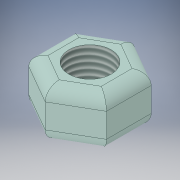
# Autodesk Inventor part: BASE_TUERCA
Saved by Autodesk Inventor 2019 (Build 230136000, 136)
## iProperties
Created: 2020-02-12
Part Number: BASE_TUERCA
Material: Genérico
Document SubType Name: Modeling
Designer: omar-
Density: 1 g/cm^3
Appearance: Valor por defecto
Author: omar-
Autodesk Inventor part; units mm, degrees
ref_plane "YZ Plane" through (0, 0, 0) normal (1, 0, 0) x (0, 1, 0)
ref_plane "XZ Plane" through (0, 0, 0) normal (0, 1, 0) x (-1, 0, 0)
ref_plane "XY Plane" through (0, 0, 0) normal (0, 0, 1) x (1, 0, 0)
sketch "Boceto1" plane through (0, 0, 0) normal (0, 1, 0) x (-1, 0, 0)
  line L0 (0, -7.3901) -> (-6.4, -3.695)
  line L1 (-6.4, -3.695) -> (-6.4, 3.695)
  line L2 (-6.4, 3.695) -> (0, 7.3901)
  line L3 (0, 7.3901) -> (6.4, 3.695)
  line L4 (6.4, 3.695) -> (6.4, -3.695)
  line L5 (6.4, -3.695) -> (0, -7.3901)
  circle A0 centre (0, 0) radius 3.5
  dimension "d0" = 6.4
  dimension "d1" = 0
  dimension "d2" = 7
  constraints: 12 end point, 2 coincident, 1 centre point, 13 other
  measures "d0" distance from line of L5 point (0, 0)
  measures "d1" horizontal distance of point (0, 0) L0.start
  measures "d2" diameter of A0
extrude "Extrusión1" add sketch "Boceto1" along normal blind 8
fillet "Empalme1" radius 2 12 edges at (3.2, 8, 5.5426) (-3.2, 8, 5.5426) (-3.2, 8, -5.5426) (3.2, 8, -5.5426) (6.4, 8, 0) (-6.4, 8, 0) (3.2, 0, 5.5426) (6.4, 0, 0) (-3.2, 0, 5.5426) (3.2, 0, -5.5426) (-3.2, 0, -5.5426) (-6.4, 0, 0)
thread "Rosca1" size "M7x1" class "6H" standard "ANSI Metric M Profile" full length
